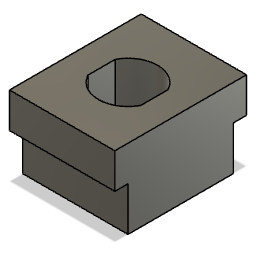
potentiometer_holder (Autodesk Fusion 360 design; units mm, degrees)
Autodesk Fusion 360 part; units mm, degrees
sketch "Sketch1" plane through (0, 0, 0) normal (0, 1, 0) x (1, 0, 0)
  line L0 (6, 6) -> (-6, 6)
  line L1 (-6, 6) -> (-6, -6)
  line L2 (-6, -6) -> (6, -6)
  line L3 (6, -6) -> (6, 6)
  line L4 (6, 6) -> (-6, -6) construction
  line L5 (-6, 6) -> (6, -6) construction
  dimension "d1" = 12
  dimension "d2" = 12
  constraint horizontal L0
  constraint perpendicular L0 L1
  constraint parallel L0 L2
  constraint parallel L1 L3
  constraint coincident L4 origin
  constraint coincident L5 origin
  measures "d1" distance of L1.end L2.end
  measures "d2" distance of L0.end L1.end
extrude "Extrude1" add sketch "Sketch1" along normal blind 4 makes body 1
sketch "Sketch2" plane through (0, 4, 0) normal (0, 1, 0) x (-1, 0, 0)
  line L0 (-6, 6) -> (-6, -6)
  line L1 (-6, -6) -> (6, -6)
  line L2 (6, -6) -> (6, 6)
  line L3 (6, 6) -> (-6, 6)
  circle A0 centre (0, 0) radius 3.375
  line L4 (-3, -3.5) -> (3, -3.5)
  line L5 (3, -3.5) -> (3, 3.5)
  line L6 (3, 3.5) -> (-3, 3.5)
  line L7 (-3, 3.5) -> (-3, -3.5)
  line L8 (-3, -3.5) -> (3, 3.5) construction
  line L9 (3, -3.5) -> (-3, 3.5) construction
  dimension "d5" = 6.75
  dimension "d6" = 6
  dimension "d7" = 7
  constraint coincident A0.centre origin
  constraint horizontal L4
  constraint perpendicular L4 L5
  constraint parallel L4 L6
  constraint parallel L5 L7
  constraint coincident L8 A0.centre
  constraint coincident L9 A0.centre
  measures "d5" diameter of A0
  measures "d6" distance of L5.end L6.end
  measures "d7" distance of L4.end L5.end
extrude "Extrude2" cut sketch "Sketch2" against normal blind 5 contours A0 L5 L7 bodies 1
sketch "Sketch3" plane through (0, 0, 0) normal (0, -1, 0) x (1, 0, 0)
  line L0 (3, 1.5462) -> (3, -1.5462)
  arc A0 (-3, -1.5462) -> (3, -1.5462) centre (0, 0) ccw
  line L1 (-3, -1.5462) -> (-3, 1.5462)
  arc A1 (3, 1.5462) -> (-3, 1.5462) centre (0, 0) ccw
  line L2 (6, -6) -> (6, 6)
  line L3 (6, 6) -> (-6, 6)
  line L4 (-6, 6) -> (-6, -6)
  line L5 (-6, -6) -> (6, -6)
  line L6 (6, 7.5) -> (-6, 7.5)
  line L7 (-6, 7.5) -> (-6, -7.5)
  line L8 (-6, -7.5) -> (6, -7.5)
  line L9 (6, -7.5) -> (6, 7.5)
  line L10 (6, 7.5) -> (-6, -7.5) construction
  line L11 (-6, 7.5) -> (6, -7.5) construction
  dimension "d10" = 12
  dimension "d11" = 15
  constraint horizontal L6
  constraint perpendicular L6 L7
  constraint parallel L6 L8
  constraint parallel L7 L9
  constraint coincident L10 A0.centre
  constraint coincident L11 A0.centre
  constraint coincident A0.centre A1.centre
  measures "d10" distance of L7.end L8.end
  measures "d11" distance of L6.end L7.end
extrude "Extrude3" add sketch "Sketch3" against normal blind 4 separate body contours L5 L7 L8 L9 | L3 L6 L7 L9 makes body 2 at (2, 1.3333, 6) makes body 3 at (-2, 1.3333, -7.5)
sketch "Sketch4" plane through (0, 0, 0) normal (0, -1, 0) x (1, 0, 0)
  line L0 (3, 1.5462) -> (3, -1.5462)
  arc A0 (-3, -1.5462) -> (3, -1.5462) centre (0, 0) ccw
  line L1 (-3, -1.5462) -> (-3, 1.5462)
  arc A1 (3, 1.5462) -> (-3, 1.5462) centre (0, 0) ccw
  line L2 (6, -6) -> (6, 6)
  line L3 (6, 6) -> (-6, 6)
  line L4 (-6, 6) -> (-6, -6)
  line L5 (-6, -6) -> (6, -6)
  line L6 (6, 6) -> (-6, 6)
  line L7 (-6, 6) -> (-6, -6)
  line L8 (-6, -6) -> (6, -6)
  line L9 (6, -6) -> (6, 6)
  line L10 (6, 6) -> (-6, -6) construction
  line L11 (-6, 6) -> (6, -6) construction
  dimension "d14" = 12
  dimension "d15" = 12
  constraint horizontal L6
  constraint perpendicular L6 L7
  constraint parallel L6 L8
  constraint parallel L7 L9
  constraint coincident L10 A0.centre
  constraint coincident L11 A0.centre
  constraint coincident A0.centre A1.centre
  measures "d14" distance of L4.end L2.start
  measures "d15" distance of L3.end L4.end
extrude "Extrude4" add sketch "Sketch4" along normal blind 5 bodies 1 2 3
sketch "Sketch5" plane through (0, -5, 0) normal (0, -1, 0) x (1, 0, 0)
  arc A0 (-3, -1.5462) -> (3, -1.5462) centre (0, 0) ccw
  line L0 (-3, -1.5462) -> (-3, 1.5462)
  arc A1 (3, 1.5462) -> (-3, 1.5462) centre (0, 0) ccw
  line L1 (3, 1.5462) -> (3, -1.5462)
  line L2 (6, -6) -> (6, 6)
  line L3 (6, 6) -> (-6, 6)
  line L4 (-6, 6) -> (-6, -6)
  line L5 (-6, -6) -> (6, -6)
  line L6 (5, 5.6) -> (-5, 5.6)
  line L7 (-5, 5.6) -> (-5, -5.6)
  line L8 (-5, -5.6) -> (5, -5.6)
  line L9 (5, -5.6) -> (5, 5.6)
  line L10 (5, 5.6) -> (-5, -5.6) construction
  line L11 (-5, 5.6) -> (5, -5.6) construction
  dimension "d18" = 11.2
  constraint horizontal L6
  constraint perpendicular L6 L7
  constraint parallel L6 L8
  constraint parallel L7 L9
  constraint coincident L10 A0.centre
  constraint coincident L11 A0.centre
  constraint coincident A0.centre A1.centre
  measures "d18" distance of L6.end L7.end
